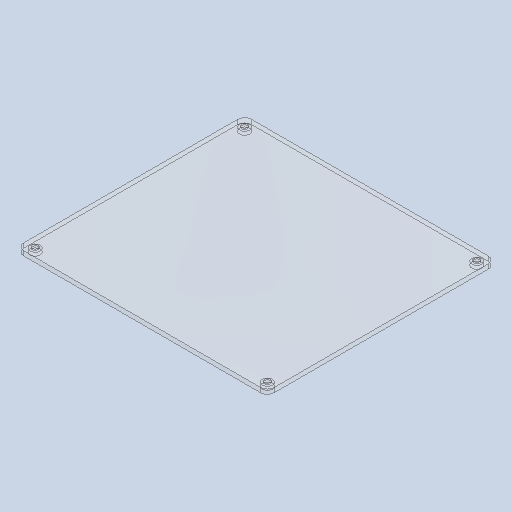
# Autodesk Inventor part: podstawa
Saved by Autodesk Inventor 2025 (Build 290162000, 162)
## iProperties
Created: 2026-04-02
Part Number: podstawa
Material: Tworzywo sztuczne PET
Document SubType Name: Modeling
Designer: zzapa
Density: 1.541 g/cm^3
Appearance: Poliwęglan — przezroczysty
Author: zzapa
Autodesk Inventor part; units mm, degrees
ref_plane "YZ Plane" through (0, 0, 0) normal (1, 0, 0) x (0, 1, 0)
ref_plane "XZ Plane" through (0, 0, 0) normal (0, 1, 0) x (-1, 0, 0)
ref_plane "XY Plane" through (0, 0, 0) normal (0, 0, 1) x (1, 0, 0)
sketch "Szkic1" plane through (0, 0, 0) normal (0, 1, 0) x (-1, 0, 0)
  line L0 (110, 0) -> (0, 0)
  line L1 (0, 0) -> (0, -100)
  line L2 (0, -100) -> (110, -100)
  line L3 (110, -100) -> (110, 0)
  dimension "d0" = 100
  dimension "d1" = 110
  constraints: 8 end point, 2 parallel, 1 coincident, 1 horizontal, 1 perpendicular
  measures "d0" distance of L2.end L0.start
  measures "d1" distance of L1.end L2.end
extrude "Gabaryt" add sketch "Szkic1" along normal blind 2
sketch "Szkic2" plane through (0, 0, 0) normal (0, 1, 0) x (1, 0, 0)
  line L0 (0, 0) -> (0, 100) projected
  line L1 (-110, 0) -> (0, 0) projected
  line L2 (-110, 100) -> (-110, 0) projected
  line L3 (0, 100) -> (-110, 100) projected
  line L4 (-110, 50) -> (0, 50)
  line L5 (-55, 100) -> (-55, 0)
  point P0 (-4, 4)
  point P1 (-106, 4)
  point P2 (-4, 96)
  point P3 (-106, 96)
  dimension "d4" = 4
  dimension "d5" = 4
  constraints: 4 end point, 4 midpoint, 3 symmetric about line
  measures "d4" distance from line of point (-4, 4) L0
  measures "d5" distance from line of L1 point (-4, 4)
hole "Otwory montażowe" at (-4, 0, -4) at (-106, 0, -4) at (-106, 0, -96) at (-4, 0, -96) direction (0, 1, 0) diameter 2.6 end through all counterbore diameter 4.5 counterbore depth 1.5
fillet "Zaokrąglenie1" radius 3 4 edges at (0, 1, 0) (-110, 1, 0) (-110, 1, -100) (0, 1, -100)
equation "\"d0\" = podstawa_a"
equation "\"d1\" = podstawa_b"
equation "\"d2\" = podstawa_wys"
equation "\"d4\" = podstawa_otwory_montazowe_poz_x"
equation "\"d5\" = podstawa_otwory_montazowe_poz_y"
equation "\"d6\" = gniazdo_M2_D2"
equation "\"d8\" = gniazdo_M2_D1"
equation "\"d9\" = gniazdo_M2_glebokosc"
equation "\"d13\" = podstawa_zaokraglenie"
equation "\"podstawa_a\" = 100"
equation "\"podstawa_b\" = 110"
equation "\"podstawa_wys\" = 2"
equation "\"podstawa_otwory_montazowe_poz_y\" = 4"
equation "\"podstawa_otwory_montazowe_poz_x\" = 4"
equation "\"gniazdo_M2_D1\" = 4.5"
equation "\"gniazdo_M2_glebokosc\" = 1.5"
equation "\"gniazdo_M2_D2\" = 2.6"
equation "\"obudowa_wys\" = 45"
equation "\"obudowa_grubosc\" = 2"
equation "\"obudowa_prowadnica_odsuniecie\" = 2"
equation "\"obudowa_prowadnica_grubosc\" = 2"
equation "\"obudowa_kontrolki_a\" = 38"
equation "\"obudowa_prowadnica_wys\" = 19"
equation "\"obudowa_otwory_montazowe_poz_y\" = 4"
equation "\"obudowa_otwory_montazowe_poz_x\" = 4"
equation "\"obudowa_otwory_montazowe_material_y\" = 8"
equation "\"obudowa_otwory_montazowe_material_x\" = 8"
equation "\"insert_D\" = 2.4"
equation "\"insert_glebokosc\" = 5.5"
equation "\"obudowa_zaokraglenie\" = 3"
equation "\"podstawa_zaokraglenie\" = 3"
equation "\"obudowa_otwory_io_wys\" = 15"
equation "\"obudowa_otwory_io_D\" = 15"
equation "\"obudowa_otwory_io1_poz\" = 55"
equation "\"obudowa_otwory_io1_wys\" = 25"
equation "\"obudowa_otwory_io1_D\" = 11.5"
equation "\"obudowa_otwory_io2_poz\" = 38"
equation "\"obudowa_otwory_io2_wys\" = 25"
equation "\"obudowa_otwory_io2_D\" = 11.5"
equation "\"obudowa_otwory_pot_D\" = 8"
equation "\"input_b\" = 14.4"
equation "\"input_wys\" = 11"
equation "\"input_a\" = 9"
equation "\"obudowa_MTS_otwor_D\" = 6.2"
equation "\"obudowa_pot_poz_y\" = 15"
equation "\"obudowa_s_poz_x\" = 78"
equation "\"obudowa_s_D\" = 6.2"
equation "\"obudowa_s_poz_y\" = 15"
equation "\"obudowa_s_rozstaw_y\" = 16"
equation "\"pcb_rozstaw_x\" = 92"
equation "\"pcb_rozstaw_y\" = 58"
equation "\"obudowa_pcb_grubosc_scianki\" = 6"
equation "\"pcb_grubosc_scianki\" = 6"
equation "\"pcb_poz_y\" = 27"
equation "\"pcb_wys_bloku\" = 35"
equation "\"obudowa_footswitch_poz_y\" = 68"
equation "\"obudowa_footswitch_poz_x\" = 35"
equation "\"obudowa_footswitch_D\" = 12.3"
equation "\"obudowa_led_indicator_D\" = 4"
equation "\"obudowa_led_indicator_poz_x\" = 55"
equation "\"obudowa_podkladka_otwory\" = 4"
